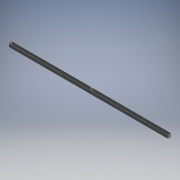
# Autodesk Inventor part: GBN1587MR3-150_info-1-16-16
Saved by Autodesk Inventor 2017.3 (Build 213256000, 256)
## iProperties
Part Number: GBN1587MR3-150_info-1-16-16
Material: Generic
Catalog Web Link: www.cadenas.de
Description: GBN__MR3-High Torque Timing Belts - MR3 Type
Vendor: MISUMI
Document SubType Name: Modeling
Designer: partserver
Manufacturer: MISUMI
Mass: 30.1504 g
Surface Area: 517.722 cm^2
Volume: 30.1504 cm^3
Density: 1 g/cm^3
Appearance: PSOLRGB-175-175-175
Category: PARTsolutions
Company: MISUMI
Title: GBN1587MR3-150
Author: Cadenas PARTsolutions
Comments: High Torque Timing Belts - MR3 Type
PSOL_IDENT_0: {$CADENAS_DATA\23d-libs\misumi\metric\48_timing_belts\gbn_mr3.prj},208 {VTYP=3D},{NB=GBN1587MR3-150_
PSOL_IDENT_1: info-1-16-16},{LINA=GBN1587MR3-150},{NN=GBN__MR3},{DATE=08.06.2021 08:28:53},{GEOMDATE=11.03.2016 00
PSOL_IDENT_2: :06:41},{VERSION=},{LINEID=40},{WBVAR=NT,RSSP,NT1,NT2},{WBNUMERIC=NT,NT1,NT2}  {NB=GBN1587MR3-150_in
PSOL_IDENT_3: fo-1-16-16},{LINA=GBN1587MR3-150},{KT=DUMMY},{PN=GBN1587MR3-150},{TYPE=GBN},{BNO=1587MR3},{BNW=15},{
PSOL_IDENT_4: BNWALG=150},{NT=529},{BC=1587},{PITCH=3},{R1=0.25},{R2=1.52},{R3=0.850},{BB=0.61},{H=2.40},{HH=1.14}
PSOL_IDENT_5: ,{II=1.26},{PLD=0.381},{RSSP=1},{RSSPALG= '1','900 or Less','2','Over 900, 1200 or Less','3','Over 1
PSOL_IDENT_6: 200, 1800 or Less','4','Over 1800, 3600 or Less','5','Over 3600, 4800 or Less' },{NT1=16},{NT1ALG=16
PSOL_IDENT_7: ,17,18,19,20,21,22,24,25,26,28,30,32,34,36,38,40,44,45,48,50,56,60,62,68,72},{NT2=16},{NT2ALG=16,17,
PSOL_IDENT_8: 18,19,20,21,22,24,25,26,28,30,32,34,36,38,40,44,45,48,50,56,60,62,68,72},{NT2ALG1=0},{NT2ALG2=16,17,
PSOL_IDENT_9: 18,19,20,21,22,24,25,26,28,30,32,34,36,38,40,44,45,48,50,56,60,62,68,72},{DRIVEP=15.27887},{DRP=14.5
PSOL_IDENT_10: 2},{DRIVENP=15.27887},{DRNP=14.52},{BBCAL=3078.00000},{C=769.50},{NOTE=-},{ASSCFGC=NT2,C},{ASSCFGCNO
PSOL_IDENT_11: TE=-},{FS=18.00},{FL=18.00},{NT1SCR=16,18,20,22,23,24,25,26,28,30,32,34,36,40,44,48,50,60},{NT2SCR=1
PSOL_IDENT_12: 6,18,20,22,23,24,25,26,28,30,32,34,36,40,44,48,50,60,72}
NB: GBN1587MR3-150_info-1-16-16
NN: GBN__MR3
NT: 529
NBSYN: $PN._info-$RSSP.-$NT1.-$NT2.
LINA: GBN1587MR3-150
CATALOG: Misumi
PN: GBN1587MR3-150
TYPE: GBN
BNO: 1587MR3
BNW: 15
BC: 1587
PITCH: 3
R1: 0.25
R2: 1.52
R3: 0.85
BB: 0.61
H: 2.4
HH: 1.14
II: 1.26
PLD: 0.381
RSSP: 900 or Less
NT1: 16
NT2: 16
SUPPLIER: MISUMI
ARTICLENO: GBN1587MR3-150_info-1-16-16
BOMINFO: GBN1587MR3-150
CREATOR: CADENAS GmbH
Autodesk Inventor part; units mm, degrees
ref_plane "YZ Plane" through (0, 0, 0) normal (1, 0, 0) x (0, 1, 0)
ref_plane "XZ Plane" through (0, 0, 0) normal (0, 1, 0) x (-1, 0, 0)
ref_plane "XY Plane" through (0, 0, 0) normal (0, 0, 1) x (1, 0, 0)
sketch "_____1" plane through (0, 0, 0) normal (0, 0, 1) x (1, 0, 0)
  arc A0 (0, 8.52) -> (0, -8.52) centre (0, 0) ccw
  line L0 (0, -8.52) -> (769.5, -8.52)
  arc A1 (769.5, -8.52) -> (769.5, 8.52) centre (769.5, 0) ccw
  line L1 (769.5, 8.52) -> (0, 8.52)
  arc A2 (0, 7.26) -> (0, -7.26) centre (0, 0) ccw
  line L2 (0, -7.26) -> (769.5, -7.26)
  arc A3 (769.5, -7.26) -> (769.5, 7.26) centre (769.5, 0) ccw
  line L3 (769.5, 7.26) -> (0, 7.26)
  constraints: 8 end point, 8 point on circle, 4 centre point
extrude "Extrusion1" add sketch "_____1" along normal mid plane 15
sketch "_____2" plane through (0, 0, 0) normal (0, 0, 1) x (1, 0, 0)
  line L0 (377.25, 8.52) -> (377.25, 7.26)
  line L1 (377.25, 7.26) -> (377.6077, 7.26)
  arc A0 (377.8552, 7.0453) -> (377.6077, 7.26) centre (377.6077, 7.01) ccw
  arc A1 (377.8552, 7.0453) -> (377.9317, 6.7401) centre (379.36, 7.26) ccw
  arc A2 (377.9317, 6.7401) -> (379.5683, 6.7401) centre (378.75, 6.97) ccw
  arc A3 (379.5683, 6.7401) -> (379.6448, 7.0453) centre (378.14, 7.26) ccw
  arc A4 (379.8923, 7.26) -> (379.6448, 7.0453) centre (379.8923, 7.01) ccw
  line L2 (379.8923, 7.26) -> (380.6077, 7.26)
  arc A5 (380.8552, 7.0453) -> (380.6077, 7.26) centre (380.6077, 7.01) ccw
  arc A6 (380.8552, 7.0453) -> (380.9317, 6.7401) centre (382.36, 7.26) ccw
  arc A7 (380.9317, 6.7401) -> (382.5683, 6.7401) centre (381.75, 6.97) ccw
  arc A8 (382.5683, 6.7401) -> (382.6448, 7.0453) centre (381.14, 7.26) ccw
  arc A9 (382.8923, 7.26) -> (382.6448, 7.0453) centre (382.8923, 7.01) ccw
  line L3 (382.8923, 7.26) -> (383.6077, 7.26)
  arc A10 (383.8552, 7.0453) -> (383.6077, 7.26) centre (383.6077, 7.01) ccw
  arc A11 (383.8552, 7.0453) -> (383.9317, 6.7401) centre (385.36, 7.26) ccw
  arc A12 (383.9317, 6.7401) -> (385.5683, 6.7401) centre (384.75, 6.97) ccw
  arc A13 (385.5683, 6.7401) -> (385.6448, 7.0453) centre (384.14, 7.26) ccw
  arc A14 (385.8923, 7.26) -> (385.6448, 7.0453) centre (385.8923, 7.01) ccw
  line L4 (385.8923, 7.26) -> (386.6077, 7.26)
  arc A15 (386.8552, 7.0453) -> (386.6077, 7.26) centre (386.6077, 7.01) ccw
  arc A16 (386.8552, 7.0453) -> (386.9317, 6.7401) centre (388.36, 7.26) ccw
  arc A17 (386.9317, 6.7401) -> (388.5683, 6.7401) centre (387.75, 6.97) ccw
  arc A18 (388.5683, 6.7401) -> (388.6448, 7.0453) centre (387.14, 7.26) ccw
  arc A19 (388.8923, 7.26) -> (388.6448, 7.0453) centre (388.8923, 7.01) ccw
  line L5 (388.8923, 7.26) -> (389.6077, 7.26)
  arc A20 (389.8552, 7.0453) -> (389.6077, 7.26) centre (389.6077, 7.01) ccw
  arc A21 (389.8552, 7.0453) -> (389.9317, 6.7401) centre (391.36, 7.26) ccw
  arc A22 (389.9317, 6.7401) -> (391.5683, 6.7401) centre (390.75, 6.97) ccw
  arc A23 (391.5683, 6.7401) -> (391.6448, 7.0453) centre (390.14, 7.26) ccw
  arc A24 (391.8923, 7.26) -> (391.6448, 7.0453) centre (391.8923, 7.01) ccw
  line L6 (391.8923, 7.26) -> (392.25, 7.26)
  line L7 (392.25, 7.26) -> (392.25, 8.52)
  line L8 (392.25, 8.52) -> (377.25, 8.52)
  constraints: 50 point on circle, 25 centre point, 18 end point
extrude "Extrusion2" add sketch "_____2" along normal mid plane 15
body "Solid1"
